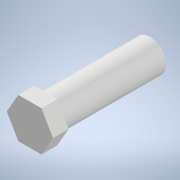
# Autodesk Inventor part: BOLT 3
Saved by Autodesk Inventor 2021 (Build 250183000, 183)
## iProperties
Created: 2021-07-27
Part Number: BOLT 3
Material: Generic
Document SubType Name: Modeling
Designer: HP
Density: 1 g/cm^3
Appearance: Default
Author: HP
Autodesk Inventor part; units mm, degrees
ref_plane "YZ Plane" through (0, 0, 0) normal (1, 0, 0) x (0, 1, 0)
ref_plane "XZ Plane" through (0, 0, 0) normal (0, 1, 0) x (-1, 0, 0)
ref_plane "XY Plane" through (0, 0, 0) normal (0, 0, 1) x (1, 0, 0)
sketch "Sketch1" plane through (0, 0, 0) normal (0, 0, 1) x (1, 0, 0)
  circle A0 centre (0, 0) radius 0.7743
  constraints: 1 centre point, 1 coincident
extrude "Extrusion1" add sketch "Sketch1" against normal blind 5.08
sketch "Sketch2" plane through (0, 0, 0) normal (0, 0, 1) x (1, 0, 0)
  circle A0 centre (0, 0) radius 0.7743 projected
  line L0 (-1.1229, 0) -> (-0.5615, 0.9725)
  line L1 (-0.5615, 0.9725) -> (0.5615, 0.9725)
  line L2 (0.5615, 0.9725) -> (1.1229, 0)
  line L3 (1.1229, 0) -> (0.5615, -0.9725)
  line L4 (0.5615, -0.9725) -> (-0.5615, -0.9725)
  line L5 (-0.5615, -0.9725) -> (-1.1229, 0)
  constraints: 12 end point, 1 coincident, 13 other
extrude "Extrusion2" add sketch "Sketch2" along normal blind 0.762 contours A0 | L0 L1 L2 L3 L4 L5
body "Solid1"
